Autodesk Fusion 360 part; units mm, degrees
note: some values were not read from the file. Chosen so that the rebuilt part matches the saved one: which bodies a step acts on. Set by a fixed rule: which sketch regions a step uses.
(part 6 of 6)
equation "d307 = -efni"
equation "d309 = bfingur_toppur"
equation "d310 = ( bfingur_toppur - pusl_fingurb ) / 2"
equation "d311 = ( bfingur_toppur - pusl_fingurb ) / 2"
equation "d312 = 2 * efni"
equation "d313 = 2 * efni"
equation "d314 = bil_milli_pusla"
equation "d315 = efni - ( bil_milli_pusla ) / 2"
equation "d319 = bil_milli_pusla / 2"
equation "d320 = efni - bil_milli_pusla / 2"
equation "d321 = ( lfingur_toppur - pusl_fingur_l ) / 2"
equation "d322 = ( lfingur_toppur - pusl_fingur_l ) / 2"
equation "d323 = efni - bil_milli_pusla / 2"
equation "d324 = lfingur_toppur"
equation "d327 = efni - bil_milli_pusla / 2"
equation "d328 = bil_milli_pusla / 2"
equation "d329 = ( bfingur_toppur - pusl_fingurb ) / 2"
equation "d330 = bfingur_toppur"
equation "d331 = efni - bil_milli_pusla / 2"
equation "d332 = ( bfingur_toppur - pusl_fingurb ) / 2"
equation "d333 = -efni"
equation "d335 = bil_milli_pusla / 2"
equation "d337 = efni - bil_milli_pusla / 2"
equation "d338 = ( bfingur_toppur - pusl_fingurb ) / 2"
equation "d339 = bfingur_toppur"
equation "d340 = ( bfingur_toppur - pusl_fingurb ) / 2"
equation "d341 = efni - bil_milli_pusla / 2"
equation "d342 = ( lfingur_toppur - pusl_fingur_l ) / 2"
equation "d343 = 2 * efni"
equation "d344 = lfingur_toppur"
equation "d345 = bil_milli_pusla"
equation "d346 = efni - bil_milli_pusla / 2"
equation "d347 = ( lfingur_toppur - pusl_fingur_l ) / 2"
equation "d348 = 2 * efni"
equation "d349 = ( bfingur_toppur - pusl_fingurb ) / 2"
equation "d350 = 2 * efni"
equation "d351 = bil_milli_pusla"
equation "d352 = bfingur_toppur"
equation "d353 = efni - bil_milli_pusla / 2"
equation "d354 = ( bfingur_toppur - pusl_fingurb ) / 2"
equation "d355 = 2 * efni"
equation "d357 = -efni"
equation "puslubil_L = ( lfingur_toppur - pusl_fingur_l ) / 2"
equation "puslubil_B = ( bfingur_toppur - pusl_fingurb ) / 2"
equation "d363 = efni - bil_milli_pusla / 2"
equation "d364 = bil_milli_pusla / 2"
equation "d365 = bfingur_toppur"
equation "d366 = puslubil_B"
equation "d367 = puslubil_B"
equation "d368 = efni - bil_milli_pusla / 2"
equation "d369 = efni - bil_milli_pusla / 2"
equation "d370 = bil_milli_pusla / 2"
equation "d371 = puslubil_L"
equation "d372 = lfingur_toppur"
equation "d373 = efni - bil_milli_pusla / 2"
equation "d374 = puslubil_L"
equation "d375 = puslubil_B"
equation "d376 = puslubil_B"
equation "d377 = 2 * efni"
equation "d378 = 2 * efni"
equation "d379 = bil_milli_pusla"
equation "d380 = efni - bil_milli_pusla / 2"
equation "d381 = bfingur_toppur"
equation "d382 = -efni"
equation "d384 = puslubil_B"
equation "d385 = puslubil_B"
equation "d386 = 2 * efni"
equation "d387 = 2 * efni"
equation "d388 = bil_milli_pusla"
equation "d389 = efni - bil_milli_pusla / 2"
equation "d391 = puslubil_L"
equation "d392 = efni - bil_milli_pusla / 2"
equation "d393 = bil_milli_pusla / 2"
equation "d394 = lfingur_toppur"
equation "d395 = puslubil_L"
equation "d396 = efni - bil_milli_pusla / 2"
equation "d397 = puslubil_L"
equation "d398 = puslubil_L"
equation "d399 = 2 * efni"
equation "d400 = 2 * efni"
equation "d401 = bil_milli_pusla"
equation "d402 = efni - bil_milli_pusla / 2"
equation "d403 = lfingur_toppur"
equation "d404 = -efni"
equation "d406 = puslubil_B"
equation "d407 = puslubil_B"
equation "d408 = 2 * efni"
equation "d409 = 2 * efni"
equation "d410 = bfingur_toppur"
equation "d411 = bil_milli_pusla"
equation "d412 = efni - bil_milli_pusla / 2"
equation "d413 = 2 * efni"
equation "d414 = puslubil_L"
equation "d415 = puslubil_L"
equation "d416 = 2 * efni"
equation "d421 = bil_milli_pusla"
equation "d422 = efni - bil_milli_pusla / 2"
equation "d423 = lfingur_toppur"
equation "d424 = -efni"
equation "d426 = puslubil_L"
equation "d427 = efni - bil_milli_pusla / 2"
equation "d428 = bil_milli_pusla / 2"
equation "d429 = lfingur_toppur"
equation "d430 = puslubil_L"
equation "d431 = efni - bil_milli_pusla / 2"
equation "d432 = puslubil_B"
equation "d433 = puslubil_B"
equation "d434 = 2 * efni"
equation "d435 = 2 * efni"
equation "d436 = efni - bil_milli_pusla / 2"
equation "d437 = bil_milli_pusla"
equation "d438 = bfingur_toppur"
equation "d439 = -efni"
equation "d441 = puslubil_L"
equation "d442 = puslubil_L"
equation "d443 = efni - bil_milli_pusla / 2"
equation "d444 = efni - bil_milli_pusla / 2"
equation "d445 = bil_milli_pusla / 2"
equation "d446 = lfingur_toppur"
equation "d447 = puslubil_L"
equation "d448 = puslubil_L"
equation "d449 = bil_milli_pusla"
equation "d450 = lfingur_toppur"
equation "d451 = efni - bil_milli_pusla / 2"
equation "d452 = 2 * efni"
equation "d453 = 2 * efni"
equation "d454 = puslubil_B"
equation "d455 = puslubil_B"
equation "d456 = efni - bil_milli_pusla / 2"
equation "d457 = efni - ( bil_milli_pusla / 2 )"
equation "d458 = bfingur_toppur"
equation "d459 = bil_milli_pusla / 2"
equation "d461 = -efni"
equation "d463 = puslubil_B"
equation "d464 = puslubil_B"
equation "d465 = efni - bil_milli_pusla / 2"
equation "d466 = bfingur_toppur"
equation "d467 = efni - bil_milli_pusla / 2"
equation "d468 = bil_milli_pusla / 2"
equation "d469 = bil_milli_pusla"
equation "d470 = 2 * efni"
equation "d471 = puslubil_L"
equation "d472 = lfingur_toppur"
equation "d473 = efni - bil_milli_pusla / 2"
equation "d474 = puslubil_L"
equation "d475 = 2 * efni"
equation "d477 = -efni"
equation "d479 = efni - bil_milli_pusla / 2"
equation "d480 = bfingur_toppur"
equation "d481 = bil_milli_pusla / 2"
equation "d482 = puslubil_B"
equation "d483 = puslubil_B"
equation "d484 = efni - bil_milli_pusla / 2"
equation "d485 = efni - bil_milli_pusla / 2"
equation "d486 = puslubil_L"
equation "d487 = puslubil_L"
equation "d488 = efni - 1 / 2 * bil_milli_pusla"
equation "d489 = 0.5 * bil_milli_pusla"
equation "d490 = lfingur_toppur"
equation "d491 = -efni"
equation "pusl_brun_l = ( got_fra_brun_lengd - efni - pusl_fingur_l ) / 2"
equation "pusl_brun_b = ( got_fra_brun_breidd - efni - pusl_fingurb ) / 2"
equation "d495 = pusl_brun_l"
equation "d496 = pusl_brun_b"
equation "d497 = bil_milli_pusla"
equation "d498 = bil_milli_pusla"
equation "d499 = bil_milli_pusla"
equation "d500 = pusl_brun_b"
equation "d501 = pusl_brun_l"
equation "d502 = bil_milli_pusla"
equation "d503 = pusl_brun_b"
equation "d504 = bil_milli_pusla"
equation "d505 = bil_milli_pusla"
equation "d506 = pusl_brun_l"
equation "d507 = pusl_brun_b"
equation "d508 = bil_milli_pusla"
equation "d509 = pusl_brun_l"
equation "d510 = bil_milli_pusla"
equation "d511 = -efni"
equation "d513 = pusl_brun_b"
equation "d514 = pusl_brun_l"
equation "d515 = pusl_brun_b"
equation "d516 = pusl_brun_l"
equation "d517 = pusl_brun_l"
equation "d518 = pusl_brun_b"
equation "d519 = pusl_brun_b"
equation "d520 = pusl_brun_l"
equation "d521 = bil_milli_pusla"
equation "d522 = bil_milli_pusla"
equation "d523 = bil_milli_pusla"
equation "d524 = bil_milli_pusla"
equation "d525 = bil_milli_pusla"
equation "d526 = bil_milli_pusla"
equation "d527 = bil_milli_pusla"
equation "d528 = bil_milli_pusla"
equation "d529 = -efni"
equation "d531 = bil_milli_pusla"
equation "d532 = bil_milli_pusla"
equation "d533 = bil_milli_pusla"
equation "d534 = bil_milli_pusla"
equation "d535 = bil_milli_pusla"
equation "d536 = bil_milli_pusla"
equation "d537 = bil_milli_pusla"
equation "d538 = bil_milli_pusla"
equation "d539 = pusl_brun_b"
equation "d540 = pusl_brun_b"
equation "d541 = pusl_brun_b"
equation "d542 = pusl_brun_b"
equation "d543 = pusl_brun_l"
equation "d544 = pusl_brun_l"
equation "d545 = pusl_brun_l"
equation "d546 = pusl_brun_l"
equation "d547 = -efni"
equation "d549 = bil_milli_pusla"
equation "d550 = bil_milli_pusla"
equation "d551 = bil_milli_pusla"
equation "d552 = bil_milli_pusla"
equation "d553 = bil_milli_pusla"
equation "d554 = bil_milli_pusla"
equation "d555 = bil_milli_pusla"
equation "d556 = bil_milli_pusla"
equation "d557 = pusl_brun_l"
equation "d558 = pusl_brun_l"
equation "d559 = pusl_brun_l"
equation "d560 = pusl_brun_l"
equation "d561 = pusl_brun_b"
equation "d562 = pusl_brun_b"
equation "d563 = pusl_brun_b"
equation "d564 = pusl_brun_b"
equation "d565 = -efni"
equation "d567 = bil_milli_pusla"
equation "d568 = bil_milli_pusla"
equation "d569 = bil_milli_pusla"
equation "d570 = bil_milli_pusla"
equation "d571 = bil_milli_pusla"
equation "d572 = bil_milli_pusla"
equation "d573 = bil_milli_pusla"
equation "d574 = bil_milli_pusla"
equation "d575 = pusl_brun_b"
equation "d576 = pusl_brun_b"
equation "d577 = pusl_brun_b"
equation "d578 = pusl_brun_b"
equation "d579 = pusl_brun_l"
equation "d580 = pusl_brun_l"
equation "d581 = pusl_brun_l"
equation "d582 = pusl_brun_l"
equation "d583 = -efni"
equation "d585 = bil_milli_pusla"
equation "d586 = bil_milli_pusla"
equation "d587 = bil_milli_pusla"
equation "d588 = bil_milli_pusla"
equation "d589 = bil_milli_pusla"
equation "d590 = bil_milli_pusla"
equation "d591 = bil_milli_pusla"
equation "d592 = bil_milli_pusla"
equation "d593 = pusl_brun_b"
equation "d594 = pusl_brun_b"
equation "d595 = pusl_brun_l"
equation "d596 = pusl_brun_l"
equation "d597 = pusl_brun_b"
equation "d598 = pusl_brun_b"
equation "d599 = pusl_brun_l"
equation "d600 = pusl_brun_l"
equation "d601 = -efni"
equation "d605 = bil_milli_pusla"
equation "d606 = bil_milli_pusla"
equation "d607 = bil_milli_pusla"
equation "d608 = bil_milli_pusla"
equation "d609 = bil_milli_pusla"
equation "d610 = bil_milli_pusla"
equation "d611 = bil_milli_pusla"
equation "d613 = bil_milli_pusla"
equation "d614 = pusl_brun_b"
equation "d615 = pusl_brun_b"
equation "d616 = pusl_brun_b"
equation "d617 = pusl_brun_b"
equation "d618 = pusl_brun_l"
equation "d619 = pusl_brun_l"
equation "d620 = pusl_brun_l"
equation "d621 = pusl_brun_l"
equation "d622 = -efni"
equation "d624 = bil_milli_pusla"
equation "d625 = bil_milli_pusla"
equation "d626 = bil_milli_pusla"
equation "d627 = bil_milli_pusla"
equation "d628 = bil_milli_pusla"
equation "d629 = bil_milli_pusla"
equation "d630 = bil_milli_pusla"
equation "d631 = bil_milli_pusla"
equation "d632 = pusl_brun_b"
equation "d633 = pusl_brun_b"
equation "d634 = pusl_brun_b"
equation "d635 = pusl_brun_b"
equation "d636 = pusl_brun_l"
equation "d637 = pusl_brun_l"
equation "d638 = pusl_brun_l"
equation "d639 = pusl_brun_l"
equation "d640 = -efni"
equation "d642 = bil_milli_pusla"
equation "d643 = bil_milli_pusla"
equation "d644 = bil_milli_pusla"
equation "d645 = bil_milli_pusla"
equation "d646 = bil_milli_pusla"
equation "d647 = bil_milli_pusla"
equation "d648 = bil_milli_pusla"
equation "d649 = bil_milli_pusla"
equation "d650 = pusl_brun_l"
equation "d651 = pusl_brun_l"
equation "d652 = pusl_brun_l"
equation "d653 = pusl_brun_l"
equation "d654 = pusl_brun_b"
equation "d655 = pusl_brun_b"
equation "d656 = pusl_brun_b"
equation "d657 = pusl_brun_b"
equation "d658 = -efni"
equation "Midja_PuslannaL = ( lengd_rammi / 3 - bil_milli_pusla ) / 2"
equation "Radius_hring = ( lengd_rammi / 3 - bil_milli_pusla ) / 4"
equation "d665 = Radius_hring * 2"
equation "d666 = Radius_hring * 2"
equation "d667 = Midja_PuslannaL"
equation "d668 = -efni"
equation "Midja_PuslannaB = ( breidd_rammi / 3 - bil_milli_pusla ) / 2"
equation "d675 = Midja_PuslannaB"
equation "d676 = 2 * Radius_hring"
equation "d677 = -efni"
equation "d679 = Radius_hring * 2"
equation "d680 = Midja_PuslannaL"
equation "d681 = Midja_PuslannaB"
equation "d682 = -efni"
equation "d684 = Midja_PuslannaB"
equation "d685 = Midja_PuslannaL"
equation "d686 = 2 * Radius_hring"
equation "d687 = Midja_PuslannaB"
equation "d688 = Midja_PuslannaL"
equation "d689 = -efni"
equation "Toppur_Botn_X = ( breidd_rammi / 3 - bil_milli_pusla ) / 10"
equation "QuarterX = Midja_PuslannaL * 0.5 * tan(60 deg)"
equation "d693 = Toppur_Botn_X / 2"
equation "d694 = Toppur_Botn_X / 2"
equation "d695 = QuarterX / 2"
equation "d696 = QuarterX / 2"
equation "d698 = Toppur_Botn_X / 2"
equation "lengd_i_midju_x = Toppur_Botn_X / sin(45 deg)"
equation "BFjarlaegd_brun_x = Midja_PuslannaB - lengd_i_midju_x / 2"
equation "d701 = BFjarlaegd_brun_x"
equation "d702 = BFjarlaegd_brun_x"
equation "d703 = Toppur_Botn_X / 2"
equation "d704 = Toppur_Botn_X / 2"
equation "d705 = QuarterX / 2"
equation "d706 = QuarterX / 2"
equation "d708 = Toppur_Botn_X / 2"
equation "d709 = Toppur_Botn_X / 2"
equation "d710 = Toppur_Botn_X / 2"
equation "d711 = QuarterX / 2"
equation "d712 = QuarterX / 2"
equation "d714 = Toppur_Botn_X / 2"
equation "d715 = Toppur_Botn_X / 2"
equation "d716 = Toppur_Botn_X / 2"
equation "d717 = QuarterX / 2"
equation "d718 = QuarterX / 2"
equation "d720 = Toppur_Botn_X / 2"
equation "d733 = Toppur_Botn_X / 2"
equation "d734 = Toppur_Botn_X / 2"
equation "d735 = QuarterX / 2"
equation "d736 = QuarterX / 2"
equation "d738 = Toppur_Botn_X / 2"
equation "d740 = -efni"
named bodies: "Rammi_lengd1", "Rammi_breidd1", "Rammi_lengd2", "Rammi_breidd2", "Millihlid_breidd_11", "Millihlid_breidd12", "Millihlid_breidd_22", "Millihlid_breidd_21", "Millihlid_lengd_11", "Millihlid_lengd_12", "Millihlid_lengd_21", "millihlid_lengd_22", "Púsl1", "Púsl2", "púsl3", "púsl4", "púsl5", "púsl6", "púsl7", "púsl8", "púsl9"
